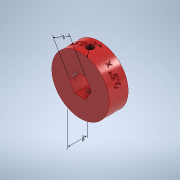
# Autodesk Inventor part: 1_2x1_2x1-1_2 HexBearing
Saved by Autodesk Inventor 2022.2 (Build 262287000, 287)
## iProperties
Created: 2020-11-08
Part Number: 1_2x1_2x1-1_2 HexBearing
Material: PC/ABS Plastic
Document SubType Name: Modeling
Designer: robst
Density: 0.357273 g/cm^3
Appearance: Red
Author: robst
Autodesk Inventor part; units mm, degrees
ref_plane "YZ Plane" through (0, 0, 0) normal (1, 0, 0) x (0, 1, 0)
sketch "Sketch1" plane through (0, 0, 0) normal (0, 0, 1) x (1, 0, 0)
  line L0 (3.6662, 6.35) -> (7.3323, 0)
  line L1 (7.3323, 0) -> (3.6662, -6.35)
  line L2 (3.6662, -6.35) -> (-3.6662, -6.35)
  line L3 (-3.6662, -6.35) -> (-7.3323, 0)
  line L4 (-7.3323, 0) -> (-3.6662, 6.35)
  line L5 (-3.6662, 6.35) -> (3.6662, 6.35)
  circle A0 centre (0, 0) radius 19.05
  circle A1 centre (0, 0) radius 7.3323 construction
  dimension "d0" = 12.7
  dimension "d2" = 38.1
  dimension "d3" = 11.7177
  constraints: 12 end point, 3 coincident, 1 centre point, 1 horizontal, 1 horizontal alignment, 15 other
  measures "d0" distance between parallel lines of L2 L5
  measures "d2" diameter of A0
extrude "Extrusion1" add sketch "Sketch1" against normal blind 12.7
ref_plane "Work Plane1" through (0, 19.05, 0) normal (0, 1, 0) x (-1, 0, 0)
sketch "Sketch2" plane through (0, 19.05, 0) normal (0, 1, 0) x (-1, 0, 0)
  line L0 (0, -6.35) -> (-25.4, -6.35) construction
  line L1 (19.05, 0) -> (-19.05, 0) construction
  spline S0 degree 2 poles (-22.7509, -6.35) (-22.7509, -7.3751) (-23.3468, -8.3353) (-23.9674, -8.3353) knots 0 0 0 1 2 2 2
  spline S1 degree 2 poles (-23.9674, -8.3353) (-24.5972, -8.3353) (-25.187, -7.3565) (-25.187, -6.3531) knots 0 0 0 1 2 2 2
  spline S2 degree 2 poles (-25.187, -6.3531) (-25.187, -5.3219) (-24.5911, -4.3678) (-23.9674, -4.3678) knots 0 0 0 1 2 2 2
  spline S3 degree 2 poles (-23.9674, -4.3678) (-23.3406, -4.3678) (-22.7509, -5.3558) (-22.7509, -6.35) knots 0 0 0 1 2 2 2
  spline S4 degree 2 poles (-23.4055, -7.5109) (-23.3314, -7.3226) (-23.2696, -6.7421) (-23.2696, -6.35) knots 0 0 0 1 2 2 2
  spline S5 degree 2 poles (-23.2696, -6.35) (-23.2696, -5.9579) (-23.3314, -5.3805) (-23.4085, -5.186) knots 0 0 0 1 2 2 2
  spline S6 degree 2 poles (-23.4085, -5.186) (-23.4857, -4.9915) (-23.7544, -4.7908) (-23.9674, -4.7908) knots 0 0 0 1 2 2 2
  spline S7 degree 2 poles (-23.9674, -4.7908) (-24.1804, -4.7908) (-24.4552, -4.9915) (-24.5355, -5.1922) knots 0 0 0 1 2 2 2
  spline S8 degree 2 poles (-24.5355, -5.1922) (-24.6127, -5.3867) (-24.6683, -5.9795) (-24.6683, -6.3531) knots 0 0 0 1 2 2 2
  spline S9 degree 2 poles (-24.6683, -6.3531) (-24.6683, -6.7545) (-24.6189, -7.2917) (-24.5386, -7.5016) knots 0 0 0 1 2 2 2
  spline S10 degree 2 poles (-24.5386, -7.5016) (-24.4645, -7.6992) (-24.1897, -7.9123) (-23.9674, -7.9123) knots 0 0 0 1 2 2 2
  spline S11 degree 2 poles (-23.9674, -7.9123) (-23.7574, -7.9123) (-23.4826, -7.7116) (-23.4055, -7.5109) knots 0 0 0 1 2 2 2
  line L2 (-21.4449, -8.255) -> (-22.0562, -8.255)
  line L3 (-22.0562, -8.255) -> (-22.0562, -7.5263)
  line L4 (-22.0562, -7.5263) -> (-21.4449, -7.5263)
  line L5 (-21.4449, -7.5263) -> (-21.4449, -8.255)
  spline S12 degree 2 poles (-18.3666, -7.0447) (-18.3666, -7.3195) (-18.5426, -7.7888) (-18.7032, -7.9617) knots 0 0 0 1 2 2 2
  spline S13 degree 2 poles (-18.7032, -7.9617) (-18.8637, -8.1346) (-19.3423, -8.3353) (-19.6387, -8.3353) knots 0 0 0 1 2 2 2
  spline S14 degree 2 poles (-19.6387, -8.3353) (-19.9104, -8.3353) (-20.4414, -8.2149) (-20.636, -8.1191) knots 0 0 0 1 2 2 2
  line L6 (-20.636, -8.1191) -> (-20.636, -7.5788)
  line L7 (-20.636, -7.5788) -> (-20.5989, -7.5788)
  spline S15 degree 2 poles (-20.5989, -7.5788) (-20.5402, -7.6221) (-20.321, -7.7332) (-20.1883, -7.7826) knots 0 0 0 1 2 2 2
  spline S16 degree 2 poles (-20.1883, -7.7826) (-20.037, -7.8351) (-19.7869, -7.8938) (-19.6294, -7.8938) knots 0 0 0 1 2 2 2
  spline S17 degree 2 poles (-19.6294, -7.8938) (-19.475, -7.8938) (-19.1848, -7.7826) (-19.0798, -7.6622) knots 0 0 0 1 2 2 2
  spline S18 degree 2 poles (-19.0798, -7.6622) (-18.9841, -7.548) (-18.8853, -7.2454) (-18.8853, -7.0416) knots 0 0 0 1 2 2 2
  spline S19 degree 2 poles (-18.8853, -7.0416) (-18.8853, -6.8378) (-18.9965, -6.5785) (-19.1015, -6.492) knots 0 0 0 1 2 2 2
  spline S20 degree 2 poles (-19.1015, -6.492) (-19.2095, -6.3963) (-19.5306, -6.316) (-19.7251, -6.316) knots 0 0 0 1 2 2 2
  spline S21 degree 2 poles (-19.7251, -6.316) (-19.9351, -6.316) (-20.3519, -6.3809) (-20.4785, -6.4087) knots 0 0 0 1 2 2 2
  line L8 (-20.4785, -6.4087) -> (-20.4785, -4.445)
  line L9 (-20.4785, -4.445) -> (-18.3882, -4.445)
  line L10 (-18.3882, -4.445) -> (-18.3882, -4.8927)
  line L11 (-18.3882, -4.8927) -> (-19.9876, -4.8927)
  line L12 (-19.9876, -4.8927) -> (-19.9876, -5.9085)
  spline S22 degree 2 poles (-19.9876, -5.9085) (-19.895, -5.8961) (-19.7159, -5.8869) (-19.6418, -5.8869) knots 0 0 0 1 2 2 2
  spline S23 degree 2 poles (-19.6418, -5.8869) (-19.3485, -5.8869) (-18.944, -5.9826) (-18.7587, -6.1246) knots 0 0 0 1 2 2 2
  spline S24 degree 2 poles (-18.7587, -6.1246) (-18.5704, -6.2666) (-18.3666, -6.6989) (-18.3666, -7.0447) knots 0 0 0 1 2 2 2
  line L13 (-16.2826, -4.2752) -> (-16.3937, -5.7572)
  line L14 (-16.3937, -5.7572) -> (-16.7302, -5.7572)
  line L15 (-16.7302, -5.7572) -> (-16.8414, -4.2752)
  line L16 (-16.8414, -4.2752) -> (-16.2826, -4.2752)
  line L17 (-17.2459, -4.2752) -> (-17.357, -5.7572)
  line L18 (-17.357, -5.7572) -> (-17.6935, -5.7572)
  line L19 (-17.6935, -5.7572) -> (-17.8047, -4.2752)
  line L20 (-17.8047, -4.2752) -> (-17.2459, -4.2752)
  line L21 (-11.7871, -8.255) -> (-12.3768, -8.255)
  line L22 (-12.3768, -8.255) -> (-13.0715, -7.1805)
  line L23 (-13.0715, -7.1805) -> (-13.7847, -8.255)
  line L24 (-13.7847, -8.255) -> (-14.3312, -8.255)
  line L25 (-14.3312, -8.255) -> (-13.3401, -6.8378)
  line L26 (-13.3401, -6.8378) -> (-14.322, -5.396)
  line L27 (-14.322, -5.396) -> (-13.7323, -5.396)
  line L28 (-13.7323, -5.396) -> (-13.0407, -6.4612)
  line L29 (-13.0407, -6.4612) -> (-12.3336, -5.396)
  line L30 (-12.3336, -5.396) -> (-11.7871, -5.396)
  line L31 (-11.7871, -5.396) -> (-12.772, -6.807)
  line L32 (-12.772, -6.807) -> (-11.7871, -8.255)
  spline S25 degree 2 poles (5.6141, -6.35) (5.6141, -7.3751) (5.0183, -8.3353) (4.3977, -8.3353) knots 0 0 0 1 2 2 2
  spline S26 degree 2 poles (4.3977, -8.3353) (3.7678, -8.3353) (3.1781, -7.3565) (3.1781, -6.3531) knots 0 0 0 1 2 2 2
  spline S27 degree 2 poles (3.1781, -6.3531) (3.1781, -5.3219) (3.774, -4.3678) (4.3977, -4.3678) knots 0 0 0 1 2 2 2
  spline S28 degree 2 poles (4.3977, -4.3678) (5.0244, -4.3678) (5.6141, -5.3558) (5.6141, -6.35) knots 0 0 0 1 2 2 2
  spline S29 degree 2 poles (4.9596, -7.5109) (5.0337, -7.3226) (5.0954, -6.7421) (5.0954, -6.35) knots 0 0 0 1 2 2 2
  spline S30 degree 2 poles (5.0954, -6.35) (5.0954, -5.9579) (5.0337, -5.3805) (4.9565, -5.186) knots 0 0 0 1 2 2 2
  spline S31 degree 2 poles (4.9565, -5.186) (4.8793, -4.9915) (4.6107, -4.7908) (4.3977, -4.7908) knots 0 0 0 1 2 2 2
  spline S32 degree 2 poles (4.3977, -4.7908) (4.1846, -4.7908) (3.9098, -4.9915) (3.8296, -5.1922) knots 0 0 0 1 2 2 2
  spline S33 degree 2 poles (3.8296, -5.1922) (3.7524, -5.3867) (3.6968, -5.9795) (3.6968, -6.3531) knots 0 0 0 1 2 2 2
  spline S34 degree 2 poles (3.6968, -6.3531) (3.6968, -6.7545) (3.7462, -7.2917) (3.8265, -7.5016) knots 0 0 0 1 2 2 2
  spline S35 degree 2 poles (3.8265, -7.5016) (3.9006, -7.6992) (4.1754, -7.9123) (4.3977, -7.9123) knots 0 0 0 1 2 2 2
  spline S36 degree 2 poles (4.3977, -7.9123) (4.6076, -7.9123) (4.8824, -7.7116) (4.9596, -7.5109) knots 0 0 0 1 2 2 2
  line L33 (6.9202, -8.255) -> (6.3088, -8.255)
  line L34 (6.3088, -8.255) -> (6.3088, -7.5263)
  line L35 (6.3088, -7.5263) -> (6.9202, -7.5263)
  line L36 (6.9202, -7.5263) -> (6.9202, -8.255)
  spline S37 degree 2 poles (9.9984, -7.0447) (9.9984, -7.3195) (9.8224, -7.7888) (9.6619, -7.9617) knots 0 0 0 1 2 2 2
  spline S38 degree 2 poles (9.6619, -7.9617) (9.5013, -8.1346) (9.0228, -8.3353) (8.7264, -8.3353) knots 0 0 0 1 2 2 2
  spline S39 degree 2 poles (8.7264, -8.3353) (8.4547, -8.3353) (7.9236, -8.2149) (7.7291, -8.1191) knots 0 0 0 1 2 2 2
  line L37 (7.7291, -8.1191) -> (7.7291, -7.5788)
  line L38 (7.7291, -7.5788) -> (7.7661, -7.5788)
  spline S40 degree 2 poles (7.7661, -7.5788) (7.8248, -7.6221) (8.044, -7.7332) (8.1768, -7.7826) knots 0 0 0 1 2 2 2
  spline S41 degree 2 poles (8.1768, -7.7826) (8.3281, -7.8351) (8.5782, -7.8938) (8.7356, -7.8938) knots 0 0 0 1 2 2 2
  spline S42 degree 2 poles (8.7356, -7.8938) (8.89, -7.8938) (9.1802, -7.7826) (9.2852, -7.6622) knots 0 0 0 1 2 2 2
  spline S43 degree 2 poles (9.2852, -7.6622) (9.3809, -7.548) (9.4797, -7.2454) (9.4797, -7.0416) knots 0 0 0 1 2 2 2
  spline S44 degree 2 poles (9.4797, -7.0416) (9.4797, -6.8378) (9.3686, -6.5785) (9.2636, -6.492) knots 0 0 0 1 2 2 2
  spline S45 degree 2 poles (9.2636, -6.492) (9.1555, -6.3963) (8.8344, -6.316) (8.6399, -6.316) knots 0 0 0 1 2 2 2
  spline S46 degree 2 poles (8.6399, -6.316) (8.43, -6.316) (8.0131, -6.3809) (7.8866, -6.4087) knots 0 0 0 1 2 2 2
  line L39 (7.8866, -6.4087) -> (7.8866, -4.445)
  line L40 (7.8866, -4.445) -> (9.9768, -4.445)
  line L41 (9.9768, -4.445) -> (9.9768, -4.8927)
  line L42 (9.9768, -4.8927) -> (8.3775, -4.8927)
  line L43 (8.3775, -4.8927) -> (8.3775, -5.9085)
  spline S47 degree 2 poles (8.3775, -5.9085) (8.4701, -5.8961) (8.6492, -5.8869) (8.7233, -5.8869) knots 0 0 0 1 2 2 2
  spline S48 degree 2 poles (8.7233, -5.8869) (9.0166, -5.8869) (9.4211, -5.9826) (9.6063, -6.1246) knots 0 0 0 1 2 2 2
  spline S49 degree 2 poles (9.6063, -6.1246) (9.7946, -6.2666) (9.9984, -6.6989) (9.9984, -7.0447) knots 0 0 0 1 2 2 2
  line L44 (12.0825, -4.2752) -> (11.9713, -5.7572)
  line L45 (11.9713, -5.7572) -> (11.6348, -5.7572)
  line L46 (11.6348, -5.7572) -> (11.5237, -4.2752)
  line L47 (11.5237, -4.2752) -> (12.0825, -4.2752)
  line L48 (11.1192, -4.2752) -> (11.008, -5.7572)
  line L49 (11.008, -5.7572) -> (10.6715, -5.7572)
  line L50 (10.6715, -5.7572) -> (10.5603, -4.2752)
  line L51 (10.5603, -4.2752) -> (11.1192, -4.2752)
  line L52 (16.5779, -8.255) -> (15.9882, -8.255)
  line L53 (15.9882, -8.255) -> (15.2935, -7.1805)
  line L54 (15.2935, -7.1805) -> (14.5803, -8.255)
  line L55 (14.5803, -8.255) -> (14.0338, -8.255)
  line L56 (14.0338, -8.255) -> (15.0249, -6.8378)
  line L57 (15.0249, -6.8378) -> (14.0431, -5.396)
  line L58 (14.0431, -5.396) -> (14.6328, -5.396)
  line L59 (14.6328, -5.396) -> (15.3244, -6.4612)
  line L60 (15.3244, -6.4612) -> (16.0314, -5.396)
  line L61 (16.0314, -5.396) -> (16.5779, -5.396)
  line L62 (16.5779, -5.396) -> (15.593, -6.807)
  line L63 (15.593, -6.807) -> (16.5779, -8.255)
  line L64 (20.6751, -8.255) -> (18.8164, -8.255)
  line L65 (18.8164, -8.255) -> (18.8164, -7.866)
  line L66 (18.8164, -7.866) -> (19.508, -7.866)
  line L67 (19.508, -7.866) -> (19.508, -5.3126)
  line L68 (19.508, -5.3126) -> (18.8164, -5.3126)
  line L69 (18.8164, -5.3126) -> (18.8164, -4.9637)
  spline S50 degree 2 poles (18.8164, -4.9637) (19.2085, -4.9637) (19.579, -4.7414) (19.6037, -4.4326) knots 0 0 0 1 2 2 2
  line L70 (19.6037, -4.4326) -> (19.9989, -4.4326)
  line L71 (19.9989, -4.4326) -> (19.9989, -7.866)
  line L72 (19.9989, -7.866) -> (20.6751, -7.866)
  line L73 (20.6751, -7.866) -> (20.6751, -8.255)
  line L74 (22.1941, -8.255) -> (21.5828, -8.255)
  line L75 (21.5828, -8.255) -> (21.5828, -7.5263)
  line L76 (21.5828, -7.5263) -> (22.1941, -7.5263)
  line L77 (22.1941, -7.5263) -> (22.1941, -8.255)
  spline S51 degree 2 poles (25.2724, -7.0447) (25.2724, -7.3195) (25.0964, -7.7888) (24.9358, -7.9617) knots 0 0 0 1 2 2 2
  spline S52 degree 2 poles (24.9358, -7.9617) (24.7753, -8.1346) (24.2967, -8.3353) (24.0003, -8.3353) knots 0 0 0 1 2 2 2
  spline S53 degree 2 poles (24.0003, -8.3353) (23.7286, -8.3353) (23.1976, -8.2149) (23.0031, -8.1191) knots 0 0 0 1 2 2 2
  line L78 (23.0031, -8.1191) -> (23.0031, -7.5788)
  line L79 (23.0031, -7.5788) -> (23.0401, -7.5788)
  spline S54 degree 2 poles (23.0401, -7.5788) (23.0988, -7.6221) (23.318, -7.7332) (23.4507, -7.7826) knots 0 0 0 1 2 2 2
  spline S55 degree 2 poles (23.4507, -7.7826) (23.602, -7.8351) (23.8521, -7.8938) (24.0096, -7.8938) knots 0 0 0 1 2 2 2
  spline S56 degree 2 poles (24.0096, -7.8938) (24.164, -7.8938) (24.4542, -7.7826) (24.5592, -7.6622) knots 0 0 0 1 2 2 2
  spline S57 degree 2 poles (24.5592, -7.6622) (24.6549, -7.548) (24.7537, -7.2454) (24.7537, -7.0416) knots 0 0 0 1 2 2 2
  spline S58 degree 2 poles (24.7537, -7.0416) (24.7537, -6.8378) (24.6425, -6.5785) (24.5376, -6.492) knots 0 0 0 1 2 2 2
  spline S59 degree 2 poles (24.5376, -6.492) (24.4295, -6.3963) (24.1084, -6.316) (23.9139, -6.316) knots 0 0 0 1 2 2 2
  spline S60 degree 2 poles (23.9139, -6.316) (23.7039, -6.316) (23.2871, -6.3809) (23.1605, -6.4087) knots 0 0 0 1 2 2 2
  line L80 (23.1605, -6.4087) -> (23.1605, -4.445)
  line L81 (23.1605, -4.445) -> (25.2508, -4.445)
  line L82 (25.2508, -4.445) -> (25.2508, -4.8927)
  line L83 (25.2508, -4.8927) -> (23.6514, -4.8927)
  line L84 (23.6514, -4.8927) -> (23.6514, -5.9085)
  spline S61 degree 2 poles (23.6514, -5.9085) (23.7441, -5.8961) (23.9231, -5.8869) (23.9972, -5.8869) knots 0 0 0 1 2 2 2
  spline S62 degree 2 poles (23.9972, -5.8869) (24.2906, -5.8869) (24.695, -5.9826) (24.8803, -6.1246) knots 0 0 0 1 2 2 2
  spline S63 degree 2 poles (24.8803, -6.1246) (25.0686, -6.2666) (25.2724, -6.6989) (25.2724, -7.0447) knots 0 0 0 1 2 2 2
  line L85 (27.3565, -4.2752) -> (27.2453, -5.7572)
  line L86 (27.2453, -5.7572) -> (26.9088, -5.7572)
  line L87 (26.9088, -5.7572) -> (26.7976, -4.2752)
  line L88 (26.7976, -4.2752) -> (27.3565, -4.2752)
  line L89 (26.3932, -4.2752) -> (26.282, -5.7572)
  line L90 (26.282, -5.7572) -> (25.9455, -5.7572)
  line L91 (25.9455, -5.7572) -> (25.8343, -4.2752)
  line L92 (25.8343, -4.2752) -> (26.3932, -4.2752)
  spline S64 degree 2 poles (32.0279, -6.7792) (32.0279, -7.48) (31.3486, -8.3353) (30.8361, -8.3353) knots 0 0 0 1 2 2 2
  spline S65 degree 2 poles (30.8361, -8.3353) (30.6045, -8.3353) (30.2742, -8.221) (30.1136, -8.1222) knots 0 0 0 1 2 2 2
  line L93 (30.1136, -8.1222) -> (30.0827, -8.255)
  line L94 (30.0827, -8.255) -> (29.632, -8.255)
  line L95 (29.632, -8.255) -> (29.632, -4.2752)
  line L96 (29.632, -4.2752) -> (30.1136, -4.2752)
  line L97 (30.1136, -4.2752) -> (30.1136, -5.6954)
  spline S66 degree 2 poles (30.1136, -5.6954) (30.2958, -5.5318) (30.7188, -5.3157) (30.9874, -5.3157) knots 0 0 0 1 2 2 2
  spline S67 degree 2 poles (30.9874, -5.3157) (31.4721, -5.3157) (32.0279, -6.0906) (32.0279, -6.7792) knots 0 0 0 1 2 2 2
  spline S68 degree 2 poles (31.5308, -6.8162) (31.5308, -6.3037) (31.2189, -5.7726) (30.8731, -5.7726) knots 0 0 0 1 2 2 2
  spline S69 degree 2 poles (30.8731, -5.7726) (30.6786, -5.7726) (30.2773, -5.9579) (30.1136, -6.0999) knots 0 0 0 1 2 2 2
  line L98 (30.1136, -6.0999) -> (30.1136, -7.7394)
  spline S70 degree 2 poles (30.1136, -7.7394) (30.2958, -7.8289) (30.5767, -7.903) (30.7435, -7.903) knots 0 0 0 1 2 2 2
  spline S71 degree 2 poles (30.7435, -7.903) (31.1109, -7.903) (31.5308, -7.3812) (31.5308, -6.8162) knots 0 0 0 1 2 2 2
  line L99 (34.7511, -8.255) -> (34.2694, -8.255)
  line L100 (34.2694, -8.255) -> (34.2694, -7.9401)
  spline S72 degree 2 poles (34.2694, -7.9401) (34.0471, -8.1346) (33.6488, -8.3353) (33.4018, -8.3353) knots 0 0 0 1 2 2 2
  spline S73 degree 2 poles (33.4018, -8.3353) (33.2166, -8.3353) (32.8862, -8.2118) (32.7658, -8.079) knots 0 0 0 1 2 2 2
  spline S74 degree 2 poles (32.7658, -8.079) (32.6423, -7.9462) (32.5064, -7.5418) (32.5064, -7.2516) knots 0 0 0 1 2 2 2
  line L101 (32.5064, -7.2516) -> (32.5064, -5.396)
  line L102 (32.5064, -5.396) -> (32.9881, -5.396)
  line L103 (32.9881, -5.396) -> (32.9881, -7.0262)
  spline S75 degree 2 poles (32.9881, -7.0262) (32.9881, -7.2546) (33.0221, -7.5541) (33.0807, -7.6653) knots 0 0 0 1 2 2 2
  spline S76 degree 2 poles (33.0807, -7.6653) (33.1394, -7.7764) (33.3401, -7.8783) (33.5284, -7.8783) knots 0 0 0 1 2 2 2
  spline S77 degree 2 poles (33.5284, -7.8783) (33.7044, -7.8783) (34.1027, -7.6776) (34.2694, -7.5325) knots 0 0 0 1 2 2 2
  line L104 (34.2694, -7.5325) -> (34.2694, -5.396)
  line L105 (34.2694, -5.396) -> (34.7511, -5.396)
  line L106 (34.7511, -5.396) -> (34.7511, -8.255)
  spline S78 degree 2 poles (36.2207, -8.3229) (35.9336, -8.3229) (35.4365, -8.1685) (35.2729, -8.0821) knots 0 0 0 1 2 2 2
  line L107 (35.2729, -8.0821) -> (35.2729, -7.5418)
  line L108 (35.2729, -7.5418) -> (35.2976, -7.5418)
  spline S79 degree 2 poles (35.2976, -7.5418) (35.3593, -7.5912) (35.526, -7.7085) (35.665, -7.7733) knots 0 0 0 1 2 2 2
  spline S80 degree 2 poles (35.665, -7.7733) (35.7854, -7.832) (36.0818, -7.9185) (36.2393, -7.9185) knots 0 0 0 1 2 2 2
  spline S81 degree 2 poles (36.2393, -7.9185) (36.3535, -7.9185) (36.6159, -7.866) (36.6777, -7.8227) knots 0 0 0 1 2 2 2
  spline S82 degree 2 poles (36.6777, -7.8227) (36.7672, -7.7641) (36.8475, -7.6313) (36.8475, -7.4955) knots 0 0 0 1 2 2 2
  spline S83 degree 2 poles (36.8475, -7.4955) (36.8475, -7.3257) (36.6622, -7.1497) (36.4245, -7.091) knots 0 0 0 1 2 2 2
  spline S84 degree 2 poles (36.4245, -7.091) (36.3319, -7.0694) (36.0355, -7.0076) (35.9089, -6.9737) knots 0 0 0 1 2 2 2
  spline S85 degree 2 poles (35.9089, -6.9737) (35.5816, -6.878) (35.2852, -6.4828) (35.2852, -6.2018) knots 0 0 0 1 2 2 2
  spline S86 degree 2 poles (35.2852, -6.2018) (35.2852, -5.8128) (35.8688, -5.328) (36.3504, -5.328) knots 0 0 0 1 2 2 2
  spline S87 degree 2 poles (36.3504, -5.328) (36.5881, -5.328) (37.0698, -5.4454) (37.2334, -5.5349) knots 0 0 0 1 2 2 2
  line L109 (37.2334, -5.5349) -> (37.2334, -6.0505)
  line L110 (37.2334, -6.0505) -> (37.2087, -6.0505)
  spline S88 degree 2 poles (37.2087, -6.0505) (37.0235, -5.9023) (36.5727, -5.7325) (36.3411, -5.7325) knots 0 0 0 1 2 2 2
  spline S89 degree 2 poles (36.3411, -5.7325) (36.1034, -5.7325) (35.7761, -5.9332) (35.7761, -6.1339) knots 0 0 0 1 2 2 2
  spline S90 degree 2 poles (35.7761, -6.1339) (35.7761, -6.316) (35.9706, -6.492) (36.1868, -6.5476) knots 0 0 0 1 2 2 2
  spline S91 degree 2 poles (36.1868, -6.5476) (36.2917, -6.5754) (36.5573, -6.631) (36.7024, -6.6649) knots 0 0 0 1 2 2 2
  spline S92 degree 2 poles (36.7024, -6.6649) (37.0173, -6.7452) (37.3384, -7.1126) (37.3384, -7.4306) knots 0 0 0 1 2 2 2
  spline S93 degree 2 poles (37.3384, -7.4306) (37.3384, -7.6159) (37.1933, -7.9432) (37.0513, -8.0636) knots 0 0 0 1 2 2 2
  spline S94 degree 2 poles (37.0513, -8.0636) (36.9, -8.1902) (36.514, -8.3229) (36.2207, -8.3229) knots 0 0 0 1 2 2 2
  line L111 (40.0307, -8.255) -> (39.5491, -8.255)
  line L112 (39.5491, -8.255) -> (39.5491, -6.6248)
  spline S95 degree 2 poles (39.5491, -6.6248) (39.5491, -6.4272) (39.512, -6.0876) (39.4565, -5.9857) knots 0 0 0 1 2 2 2
  spline S96 degree 2 poles (39.4565, -5.9857) (39.3978, -5.8776) (39.1878, -5.7726) (39.0088, -5.7726) knots 0 0 0 1 2 2 2
  spline S97 degree 2 poles (39.0088, -5.7726) (38.8297, -5.7726) (38.4499, -5.9641) (38.2678, -6.1184) knots 0 0 0 1 2 2 2
  line L113 (38.2678, -6.1184) -> (38.2678, -8.255)
  line L114 (38.2678, -8.255) -> (37.7861, -8.255)
  line L115 (37.7861, -8.255) -> (37.7861, -4.2752)
  line L116 (37.7861, -4.2752) -> (38.2678, -4.2752)
  line L117 (38.2678, -4.2752) -> (38.2678, -5.714)
  spline S98 degree 2 poles (38.2678, -5.714) (38.4839, -5.5195) (38.9007, -5.3157) (39.1353, -5.3157) knots 0 0 0 1 2 2 2
  spline S99 degree 2 poles (39.1353, -5.3157) (39.5553, -5.3157) (40.0307, -5.8714) (40.0307, -6.3994) knots 0 0 0 1 2 2 2
  line L118 (40.0307, -6.3994) -> (40.0307, -8.255)
  line L119 (41.1978, -8.255) -> (40.7162, -8.255)
  line L120 (40.7162, -8.255) -> (40.7162, -5.396)
  line L121 (40.7162, -5.396) -> (41.1978, -5.396)
  line L122 (41.1978, -5.396) -> (41.1978, -8.255)
  line L123 (41.2318, -4.9205) -> (40.6853, -4.9205)
  line L124 (40.6853, -4.9205) -> (40.6853, -4.4203)
  line L125 (40.6853, -4.4203) -> (41.2318, -4.4203)
  line L126 (41.2318, -4.4203) -> (41.2318, -4.9205)
  line L127 (44.1495, -8.255) -> (43.6678, -8.255)
  line L128 (43.6678, -8.255) -> (43.6678, -6.6248)
  spline S100 degree 2 poles (43.6678, -6.6248) (43.6678, -6.4272) (43.6308, -6.0876) (43.5752, -5.9857) knots 0 0 0 1 2 2 2
  spline S101 degree 2 poles (43.5752, -5.9857) (43.5165, -5.8776) (43.3066, -5.7726) (43.1275, -5.7726) knots 0 0 0 1 2 2 2
  spline S102 degree 2 poles (43.1275, -5.7726) (42.9484, -5.7726) (42.5687, -5.9641) (42.3865, -6.1184) knots 0 0 0 1 2 2 2
  line L129 (42.3865, -6.1184) -> (42.3865, -8.255)
  line L130 (42.3865, -8.255) -> (41.9049, -8.255)
  line L131 (41.9049, -8.255) -> (41.9049, -5.396)
  line L132 (41.9049, -5.396) -> (42.3865, -5.396)
  line L133 (42.3865, -5.396) -> (42.3865, -5.714)
  spline S103 degree 2 poles (42.3865, -5.714) (42.6026, -5.5195) (43.0194, -5.3157) (43.2541, -5.3157) knots 0 0 0 1 2 2 2
  spline S104 degree 2 poles (43.2541, -5.3157) (43.674, -5.3157) (44.1495, -5.8714) (44.1495, -6.3994) knots 0 0 0 1 2 2 2
  line L134 (44.1495, -6.3994) -> (44.1495, -8.255)
  spline S105 degree 2 poles (44.9275, -8.712) (44.9769, -8.7336) (45.1653, -8.8015) (45.2857, -8.8293) knots 0 0 0 1 2 2 2
  spline S106 degree 2 poles (45.2857, -8.8293) (45.4185, -8.8632) (45.6438, -8.9034) (45.7766, -8.9034) knots 0 0 0 1 2 2 2
  spline S107 degree 2 poles (45.7766, -8.9034) (45.9989, -8.9034) (46.3077, -8.7861) (46.3941, -8.6811) knots 0 0 0 1 2 2 2
  spline S108 degree 2 poles (46.3941, -8.6811) (46.4775, -8.5761) (46.5423, -8.3013) (46.5423, -8.1253) knots 0 0 0 1 2 2 2
  line L135 (46.5423, -8.1253) -> (46.5423, -7.8752)
  spline S109 degree 2 poles (46.5423, -7.8752) (46.3478, -8.045) (45.9742, -8.2056) (45.6932, -8.2056) knots 0 0 0 1 2 2 2
  spline S110 degree 2 poles (45.6932, -8.2056) (45.2054, -8.2056) (44.628, -7.48) (44.628, -6.7977) knots 0 0 0 1 2 2 2
  spline S111 degree 2 poles (44.628, -6.7977) (44.628, -6.4426) (44.8287, -5.893) (44.9955, -5.6985) knots 0 0 0 1 2 2 2
  spline S112 degree 2 poles (44.9955, -5.6985) (45.156, -5.5164) (45.5975, -5.3157) (45.8322, -5.3157) knots 0 0 0 1 2 2 2
  spline S113 degree 2 poles (45.8322, -5.3157) (46.0545, -5.3157) (46.3787, -5.4207) (46.5423, -5.5164) knots 0 0 0 1 2 2 2
  line L136 (46.5423, -5.5164) -> (46.5701, -5.396)
  line L137 (46.5701, -5.396) -> (47.024, -5.396)
  line L138 (47.024, -5.396) -> (47.024, -7.9277)
  spline S114 degree 2 poles (47.024, -7.9277) (47.024, -8.6564) (46.391, -9.3356) (45.7396, -9.3356) knots 0 0 0 1 2 2 2
  spline S115 degree 2 poles (45.7396, -9.3356) (45.5296, -9.3356) (45.0912, -9.2677) (44.9028, -9.2121) knots 0 0 0 1 2 2 2
  line L139 (44.9028, -9.2121) -> (44.9028, -8.712)
  line L140 (44.9028, -8.712) -> (44.9275, -8.712)
  line L141 (46.5423, -7.48) -> (46.5423, -5.9085)
  spline S116 degree 2 poles (46.5423, -5.9085) (46.3632, -5.822) (46.0607, -5.7479) (45.9094, -5.7479) knots 0 0 0 1 2 2 2
  spline S117 degree 2 poles (45.9094, -5.7479) (45.545, -5.7479) (45.1251, -6.2852) (45.1251, -6.7884) knots 0 0 0 1 2 2 2
  spline S118 degree 2 poles (45.1251, -6.7884) (45.1251, -7.2639) (45.4432, -7.761) (45.8013, -7.761) knots 0 0 0 1 2 2 2
  spline S119 degree 2 poles (45.8013, -7.761) (45.9896, -7.761) (46.3848, -7.6128) (46.5423, -7.48) knots 0 0 0 1 2 2 2
  spline S120 degree 2 poles (66.4815, -6.7483) (66.4815, -7.4646) (65.7992, -8.3106) (65.2774, -8.3106) knots 0 0 0 1 2 2 2
  spline S121 degree 2 poles (65.2774, -8.3106) (65.0643, -8.3106) (64.7371, -8.2118) (64.5673, -8.1099) knots 0 0 0 1 2 2 2
  line L142 (64.5673, -8.1099) -> (64.5673, -9.3078)
  line L143 (64.5673, -9.3078) -> (64.0856, -9.3078)
  line L144 (64.0856, -9.3078) -> (64.0856, -5.396)
  line L145 (64.0856, -5.396) -> (64.5673, -5.396)
  line L146 (64.5673, -5.396) -> (64.5673, -5.6954)
  spline S122 degree 2 poles (64.5673, -5.6954) (64.7463, -5.5318) (65.1848, -5.3157) (65.441, -5.3157) knots 0 0 0 1 2 2 2
  spline S123 degree 2 poles (65.441, -5.3157) (65.9319, -5.3157) (66.4815, -6.0937) (66.4815, -6.7483) knots 0 0 0 1 2 2 2
  spline S124 degree 2 poles (65.9844, -6.8039) (65.9844, -6.3129) (65.6726, -5.7726) (65.3237, -5.7726) knots 0 0 0 1 2 2 2
  spline S125 degree 2 poles (65.3237, -5.7726) (65.1199, -5.7726) (64.7371, -5.9548) (64.5673, -6.0968) knots 0 0 0 1 2 2 2
  line L147 (64.5673, -6.0968) -> (64.5673, -7.7209)
  spline S126 degree 2 poles (64.5673, -7.7209) (64.7556, -7.8104) (65.0242, -7.8783) (65.1971, -7.8783) knots 0 0 0 1 2 2 2
  spline S127 degree 2 poles (65.1971, -7.8783) (65.5707, -7.8783) (65.9844, -7.3287) (65.9844, -6.8039) knots 0 0 0 1 2 2 2
  line L148 (69.2263, -5.396) -> (68.1488, -8.255)
  line L149 (68.1488, -8.255) -> (67.7165, -8.255)
  line L150 (67.7165, -8.255) -> (66.6482, -5.396)
  line L151 (66.6482, -5.396) -> (67.17, -5.396)
  line L152 (67.17, -5.396) -> (67.9512, -7.5974)
  line L153 (67.9512, -7.5974) -> (68.7261, -5.396)
  line L154 (68.7261, -5.396) -> (69.2263, -5.396)
  spline S128 degree 2 poles (71.8909, -6.35) (71.8909, -7.3751) (71.295, -8.3353) (70.6744, -8.3353) knots 0 0 0 1 2 2 2
  spline S129 degree 2 poles (70.6744, -8.3353) (70.0445, -8.3353) (69.4548, -7.3565) (69.4548, -6.3531) knots 0 0 0 1 2 2 2
  spline S130 degree 2 poles (69.4548, -6.3531) (69.4548, -5.3219) (70.0507, -4.3678) (70.6744, -4.3678) knots 0 0 0 1 2 2 2
  spline S131 degree 2 poles (70.6744, -4.3678) (71.3011, -4.3678) (71.8909, -5.3558) (71.8909, -6.35) knots 0 0 0 1 2 2 2
  spline S132 degree 2 poles (71.2363, -7.5109) (71.3104, -7.3226) (71.3721, -6.7421) (71.3721, -6.35) knots 0 0 0 1 2 2 2
  spline S133 degree 2 poles (71.3721, -6.35) (71.3721, -5.9579) (71.3104, -5.3805) (71.2332, -5.186) knots 0 0 0 1 2 2 2
  spline S134 degree 2 poles (71.2332, -5.186) (71.156, -4.9915) (70.8874, -4.7908) (70.6744, -4.7908) knots 0 0 0 1 2 2 2
  spline S135 degree 2 poles (70.6744, -4.7908) (70.4613, -4.7908) (70.1865, -4.9915) (70.1063, -5.1922) knots 0 0 0 1 2 2 2
  spline S136 degree 2 poles (70.1063, -5.1922) (70.0291, -5.3867) (69.9735, -5.9795) (69.9735, -6.3531) knots 0 0 0 1 2 2 2
  spline S137 degree 2 poles (69.9735, -6.3531) (69.9735, -6.7545) (70.0229, -7.2917) (70.1032, -7.5016) knots 0 0 0 1 2 2 2
  spline S138 degree 2 poles (70.1032, -7.5016) (70.1773, -7.6992) (70.4521, -7.9123) (70.6744, -7.9123) knots 0 0 0 1 2 2 2
  spline S139 degree 2 poles (70.6744, -7.9123) (70.8843, -7.9123) (71.1591, -7.7116) (71.2363, -7.5109) knots 0 0 0 1 2 2 2
  line L155 (74.5369, -8.255) -> (72.6782, -8.255)
  line L156 (72.6782, -8.255) -> (72.6782, -7.866)
  line L157 (72.6782, -7.866) -> (73.3698, -7.866)
  line L158 (73.3698, -7.866) -> (73.3698, -5.3126)
  line L159 (73.3698, -5.3126) -> (72.6782, -5.3126)
  line L160 (72.6782, -5.3126) -> (72.6782, -4.9637)
  spline S140 degree 2 poles (72.6782, -4.9637) (73.0703, -4.9637) (73.4408, -4.7414) (73.4655, -4.4326) knots 0 0 0 1 2 2 2
  line L161 (73.4655, -4.4326) -> (73.8607, -4.4326)
  line L162 (73.8607, -4.4326) -> (73.8607, -7.866)
  line L163 (73.8607, -7.866) -> (74.5369, -7.866)
  line L164 (74.5369, -7.866) -> (74.5369, -8.255)
  point P0 (0, 0)
  dimension "d17" = 25.4
  dimension "d18" = 6.35
  constraints: 2 end point, 2 horizontal
  measures "d17" distance of L0.start L0.end
  measures "d18" distance between parallel lines of L0 L1
emboss "Emboss1" sketch "Sketch2" operation cut depth 2.54 direction (0, -1, 0) wrap yes faces at (18.9882, -1.5329, -8.4667)
sketch "Sketch3" plane through (0, 19.05, 0) normal (0, 1, 0) x (-1, 0, 0)
  line L0 (3.6662, 0) -> (-3.6662, 0) construction
  line L1 (0, 0) -> (0, -12.7) construction
  line L2 (-3.6662, -12.7) -> (3.6662, -12.7) construction
  line L3 (19.05, 0) -> (-19.05, 0) projected
  line L4 (-19.05, -12.7) -> (19.05, -12.7) projected
  point P0 (0, 0)
  point P1 (0, -6.35)
  dimension "d28" = 6.35
  dimension "d29" = 6.35
  constraints: 3 midpoint, 2 end point
  measures "d28" distance from line of L3 point (0, -6.35)
  measures "d29" distance from line of L4 point (0, -6.35)
hole "Hole1" at (0, 19.05, -6.35) direction (0, -1, 0) diameter 4.318 end through all clearance for "Hex Machine Screw" size "#6" standard "Ansi Unified Screw Threads"
sketch "Sketch4" plane through (0, 19.05, 0) normal (0, 1, 0) x (-1, 0, 0)
  circle A0 centre (0, -6.35) radius 2.159 projected
  circle A1 centre (0, -6.35) radius 2.4257
  point P0 (0, 0)
  point P1 (0, -4.445)
  point P2 (2.0138, -5.8255)
  point P3 (2.0136, -7.3829)
  point P4 (1.4342, -8.2178)
  point P5 (-0.3417, -8.7358)
  point P6 (1.6461, -8.001)
  point P7 (1.1668, -8.4205)
  point P8 (1.1668, -4.7875)
  point P9 (1.6461, -5.207)
  point P10 (1.0457, -8.4928)
  point P11 (0.14, -8.7585)
  point P12 (2.125, -6.2226)
  point P13 (-1.8043, -5.4183)
  point P14 (2.1178, -5.9301)
  point P15 (0.2089, -4.2011)
  point P16 (2.1178, -5.9301)
  point P17 (0, -8.763)
  point P18 (0, -4.4768)
  point P19 (0, -8.7948)
  point P20 (-1.5869, -7.8139)
  point P21 (1.9368, -5.396)
  point P22 (-1.8104, -7.5263)
  point P23 (-1.5248, -4.8215)
  point P24 (1.016, -8.255)
  point P25 (-1.2608, -8.1026)
  point P26 (0.9915, -8.2679)
  dimension "d30" = 4.8514
  constraints: 1 centre point, 1 coincident, 7 other
  measures "d30" diameter of A1
extrude "Extrusion2" cut sketch "Sketch4" against normal blind 5.5524 contours A0 | A1
ref_plane "Work Plane2" through (0, -19.05, 0) normal (0, 1, 0) x (-1, 0, 0)
sketch "Sketch5" plane through (0, -19.05, 0) normal (0, 1, 0) x (-1, 0, 0)
  circle A0 centre (0, -6.35) radius 2.159 projected
  circle A1 centre (0, -6.35) radius 3.429
  point P0 (0, 0)
  point P1 (0.9744, -4.4234)
  point P2 (1.04, -8.242)
  point P3 (-2.159, -6.35)
  point P4 (1.525, -7.8783)
  point P5 (1.9368, -5.396)
  point P6 (-1.9313, -5.3848)
  point P7 (-2.159, -6.35)
  point P8 (-2.159, -6.35)
  point P9 (-2.159, -6.35)
  point P10 (-2.159, -6.35)
  point P11 (-2.159, -6.35)
  point P12 (-2.159, -6.35)
  point P13 (-2.159, -6.35)
  point P14 (-2.159, -6.35)
  point P15 (0.9925, -4.4326)
  point P16 (1.016, -8.255)
  point P17 (-1.0545, -8.234)
  point P18 (-2.159, -6.35)
  point P19 (1.2822, -8.087)
  point P20 (1.5372, -7.866)
  point P21 (1.8934, -5.3126)
  point P22 (2.1589, -6.3317)
  point P23 (-1.6556, -4.9643)
  point P24 (-1.9898, -5.5123)
  point P25 (1.5802, -7.8211)
  point P26 (1.8228, -7.507)
  dimension "d33" = 6.858
  constraints: 1 centre point, 1 coincident, 1 other
  measures "d33" diameter of A1
extrude "Extrusion3" cut sketch "Sketch5" along normal blind 1.8542 contours A0 | A1
equation "\"d0\" = hexSize"
equation "\"d2\" = externalDiameter"
equation "\"d4\" = thickness"
equation "\"hexSize\" = 12.7"
equation "\"externalDiameter\" = 38.1"
equation "\"thickness\" = 12.7"
body "Solid1"
